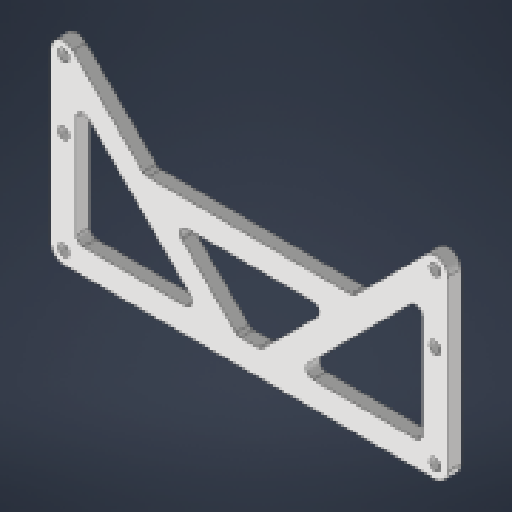
# Autodesk Inventor part: hoodbrace
Saved by Autodesk Inventor 2025.2 (Build 292293000, 293)
## iProperties
Created: 2025-12-05
Part Number: hoodbrace
Material: Generic
Document SubType Name: Modeling
Designer: cloudy
Density: 1 g/cm^3
Appearance: Default
Author: cloudy
Autodesk Inventor part; units mm, degrees
ref_plane "YZ Plane" through (0, 0, 0) normal (1, 0, 0) x (0, 1, 0)
ref_plane "XZ Plane" through (0, 0, 0) normal (0, 1, 0) x (-1, 0, 0)
ref_plane "XY Plane" through (0, 0, 0) normal (0, 0, 1) x (1, 0, 0)
sketch "Sketch1" plane through (0, 0, 0) normal (0, 0, 1) x (1, 0, 0)
  circle A0 centre (-12.7, -31.75) radius 2.1844 projected
  circle A1 centre (127, -31.75) radius 2.1844 projected
  circle A2 centre (-12.7, -95.25) radius 2.1844 projected
  circle A3 centre (127, -95.25) radius 2.1844 projected
  arc A4 (-17.4625, -95.25) -> (-12.7, -100.0125) centre (-12.7, -95.25) ccw
  arc A5 (-9.3324, -28.3824) -> (-17.4625, -31.75) centre (-12.7, -31.75) ccw
  arc A6 (131.7625, -31.75) -> (123.6324, -28.3824) centre (127, -31.75) ccw
  arc A7 (127, -100.0125) -> (131.7625, -95.25) centre (127, -95.25) ccw
  line L0 (-17.4625, -31.75) -> (-17.4625, -95.25)
  line L1 (-12.7, -100.0125) -> (127, -100.0125)
  line L2 (131.7625, -95.25) -> (131.7625, -31.75)
  line L3 (39.3023, -90.4875) -> (-7.9375, -43.2477)
  line L4 (-7.9375, -43.2477) -> (-7.9375, -90.4875)
  line L5 (122.2375, -43.2477) -> (122.2375, -90.4875)
  line L6 (122.2375, -43.2477) -> (74.9977, -90.4875)
  line L7 (57.15, -100.0125) -> (57.15, -90.4875) construction
  line L8 (-7.9375, -90.4875) -> (39.3023, -90.4875)
  line L9 (52.7727, -90.4875) -> (61.5273, -90.4875)
  line L10 (74.9977, -90.4875) -> (122.2375, -90.4875)
  line L11 (86.9273, -65.0875) -> (27.3727, -65.0875)
  line L12 (96.4523, -55.5625) -> (17.8477, -55.5625)
  line L13 (61.5273, -90.4875) -> (86.9273, -65.0875)
  line L14 (96.4523, -55.5625) -> (123.6324, -28.3824)
  line L15 (-9.3324, -28.3824) -> (17.8477, -55.5625)
  line L16 (27.3727, -65.0875) -> (52.7727, -90.4875)
  circle A8 centre (-12.7, -57.15) radius 2.1844 projected
  circle A9 centre (127, -57.15) radius 2.1844 projected
  point P0 (0, 0)
  dimension "d0" = 9.525
  dimension "d8" = 9.525
  dimension "d9" = 25.4
  dimension "d10" = 45
  constraints: 34 end point, 16 tangent, 8 point on circle, 5 horizontal, 5 parallel, 4 centre point, 4 coincident, 3 equal radius, 2 midpoint, 2 perpendicular, 2 vertical
  measures "d0" diameter of A4
  measures "d8" distance between parallel lines of L12 L11
  measures "d9" distance between parallel lines of L11 L9
  measures "d10" angle of L5 L6
extrude "Extrusion1" add sketch "Sketch1" along normal blind 5.08
fillet "Fillet2" radius 2.54 6 edges at (39.3023, -90.4875, 2.54) (74.9977, -90.4875, 2.54) (122.2375, -43.2477, 2.54) (122.2375, -90.4875, 2.54) (-7.9375, -43.2477, 2.54) (-7.9375, -90.4875, 2.54)
fillet "Fillet3" radius 2.54 6 edges at (27.3727, -65.0875, 2.54) (86.9273, -65.0875, 2.54) (96.4523, -55.5625, 2.54) (17.8477, -55.5625, 2.54) (61.5273, -90.4875, 2.54) (52.7727, -90.4875, 2.54)
body "Solid1"
